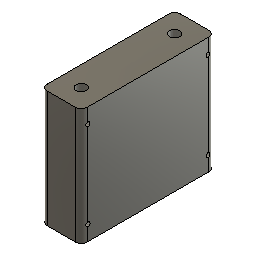
Base Spacer v8 (Autodesk Fusion 360 design; units mm, degrees)
Autodesk Fusion 360 part; units mm, degrees
sketch "Sketch1" plane through (0, 0, 0) normal (0, 1, 0) x (1, 0, 0)
  line L0 (-12, 40) -> (12, 40)
  line L1 (12, 40) -> (12, -40)
  line L2 (12, -40) -> (-12, -40)
  line L3 (-12, -40) -> (-12, 40)
  line L4 (-50, 0) -> (40, 0) construction
  line L5 (0, 60) -> (0, -56.3927) construction
  circle A0 centre (0, -28) radius 3.1
  circle A1 centre (0, 28) radius 3.1
  dimension "d1" = 24
  dimension "d2" = 80
  dimension "d3" = 12
  dimension "d4" = 40
  dimension "d5" = 6.2
  dimension "d6" = 12
  dimension "d7" = 12
  constraint horizontal L0
  constraint vertical L1
  constraint horizontal L2
  constraint vertical L3
  constraint horizontal L4
  constraint perpendicular L2 L5
  constraint symmetric L4 A0 A1
  measures "d1" distance of L0.start L0.end
  measures "d2" distance of L0.start L2.end
  measures "d3" distance of L3 L5
  measures "d4" distance of L0 L4
  measures "d5" diameter of A0
  measures "d6" distance of L3 A0.centre
  measures "d7" distance of L2 A0.centre
extrude "Extrude1" add sketch "Sketch1" along normal blind 70
fillet "Fillet1" radius 3.5 4 edges at (-12, 35, 40) (-12, 35, -40) (12, 35, -40) (12, 35, 40)
sketch "Sketch3" plane through (12, 0, 0) normal (1, 0, 0) x (0, 0, -1)
  line L0 (-36.5, 70) -> (-36.5, 0)
  line L1 (-36.5, 0) -> (36.5, 0)
  line L2 (36.5, 0) -> (36.5, 70)
  line L3 (36.5, 70) -> (-36.5, 70)
  line L4 (36, 9) -> (-36, 9)
  line L5 (-36, 9) -> (-36, 61)
  line L6 (-36, 61) -> (36, 61)
  line L7 (36, 61) -> (36, 9)
  line L8 (36, 9) -> (-36, 61) construction
  line L9 (-36, 9) -> (36, 61) construction
  circle A0 centre (-36, 61) radius 1.25
  circle A1 centre (36, 61) radius 1.25
  circle A2 centre (-36, 9) radius 1.25
  circle A3 centre (36, 9) radius 1.25
  point P0 (0, 35)
  dimension "d12" = 72
  dimension "d13" = 52
  dimension "d14" = 36.5
  dimension "d15" = 73
  dimension "d16" = 2.5
  dimension "d17" = 2.5
  dimension "d18" = 2.5
  dimension "d19" = 2.5
  dimension "d20" = 70
  dimension "d21" = 35
  constraint horizontal L4
  constraint perpendicular L4 L5
  constraint parallel L4 L6
  constraint parallel L5 L7
  constraint coincident L8 P0
  constraint coincident L9 P0
  constraint coincident L5.end L6.start
  constraint coincident L6.end L7.start
  constraint coincident L4.end L5.start
  constraint coincident L4.start L7.end
  measures "d12" distance of L5.end L6.end
  measures "d13" distance of L4.end L5.end
  measures "d14" distance of L0 P0
  measures "d15" distance of L0.start L2.end
  measures "d16" diameter of A0
  measures "d17" diameter of A1
  measures "d18" diameter of A2
  measures "d19" diameter of A3
  measures "d20" distance of L1 L3
  measures "d21" distance of L3 P0
extrude "Extrude2" cut sketch "Sketch3" against normal blind 24 contours L0 L5 L6 A0 | L0 A0 | L5 L6 A0 | L2 A1 | L2 L6 L7 A1 | L0 L4 L5 A2 | L0 A2 | L6 L7 A1 | L4 L5 A2 | L2 A3 | L2 L4 L7 A3 | L4 L7 A3
equation "d3 = d1 / 2"
equation "d4 = d2 / 2"
equation "d7 = d6"
equation "d14 = d15 / 2"
equation "d17 = d16"
equation "d18 = d16"
equation "d19 = d16"
equation "d21 = d20 / 2"
